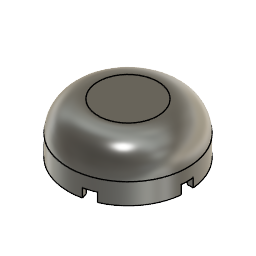
FlowerNubV0_v13 (Autodesk Fusion 360 design; units mm, degrees)
Autodesk Fusion 360 part; units mm, degrees
sketch "Sketch1" plane through (0, 0, 0) normal (0, 0, 1) x (1, 0, 0)
  circle A0 centre (0, 0) radius 3
  circle A1 centre (0, 0) radius 20
  dimension "d1" = 6
  dimension "d2" = 40
  constraint coincident A0.centre A1.centre
  constraint concentric A0 A1
  measures "d1" diameter of A0
  measures "d2" diameter of A1
extrude "Extrude1" add sketch "Sketch1" along normal blind 17 contours A0 | A1
fillet "Fillet1" radius 10 1 edges at (-18.6465, -7.2323, 17)
shell "Shell1" thickness 2 removed faces 1 at (4.7423, -7.1112, 0)
sketch "Sketch3" plane through (0, 0, 0) normal (0, 0, -1) x (1, 0, 0)
  circle A0 centre (0, 0) radius 18
  circle A1 centre (0, 0) radius 20
  line L0 (0, 0) -> (22, 0)
  line L1 (22, 0) -> (22, 2)
  line L2 (22, 0) -> (22, -2)
  line L3 (22, 2) -> (15, 2)
  line L4 (15, 2) -> (15, -2)
  line L5 (15, -2) -> (22, -2)
  line L6 (22, -2) -> (22, 2)
  line L7 (4.8963, 21.5413) -> (2.7331, 14.8839)
  line L8 (8.7005, 20.3052) -> (4.8963, 21.5413)
  line L9 (6.5374, 13.6478) -> (8.7005, 20.3052)
  line L10 (2.7331, 14.8839) -> (6.5374, 13.6478)
  line L11 (-18.9739, 11.3132) -> (-13.3108, 7.1987)
  line L12 (-16.6228, 14.5493) -> (-18.9739, 11.3132)
  line L13 (-10.9597, 10.4348) -> (-16.6228, 14.5493)
  line L14 (-13.3108, 7.1987) -> (-10.9597, 10.4348)
  line L15 (-16.6228, -14.5493) -> (-10.9597, -10.4348)
  line L16 (-18.9739, -11.3132) -> (-16.6228, -14.5493)
  line L17 (-13.3108, -7.1987) -> (-18.9739, -11.3132)
  line L18 (-10.9597, -10.4348) -> (-13.3108, -7.1987)
  line L19 (8.7005, -20.3052) -> (6.5374, -13.6478)
  line L20 (4.8963, -21.5413) -> (8.7005, -20.3052)
  line L21 (2.7331, -14.8839) -> (4.8963, -21.5413)
  line L22 (6.5374, -13.6478) -> (2.7331, -14.8839)
  dimension "d11" = 2
  dimension "d12" = 2
  dimension "d14" = 360
  constraint coincident A0.centre A1.centre
  constraint horizontal L0
  constraint perpendicular L0 L1
  constraint perpendicular L0 L2
  constraint horizontal L3
  constraint vertical L4
  constraint horizontal L5
  constraint vertical L6
  measures "d11" distance of L0.end L1.end
  measures "d12" distance of L0.end L2.end
extrude "Extrude3" cut sketch "Sketch3" against normal blind 3 contours A0 L0 L3 L4 | A0 A1 L0 L5 | A0 A1 L0 L3 | A0 L0 L4 L5 | A1 L0 L2 L5 L6 | A1 L0 L1 L3 L6 | A0 L7 L9 L10 | A0 A1 L7 L9 | A0 A1 L19 L21 | A0 L19 L21 L22 | A1 L7 L8 L9 | A1 L19 L20 L21 | A0 L11 L13 L14 | A0 A1 L11 L13 | A0 A1 L15 L17 | A0 L15 L17 L18 | A1 L11 L12 L13 | A1 L15 L16 L17
chamfer "Chamfer1" distance 2 angle 45 5 edges at (-14.5623, -10.5801, 3) (-14.5623, 10.5801, 3) (5.5623, 17.119, 3) (18, 0, 3) (5.5623, -17.119, 3) tangent chain off
sketch "Sketch2" plane through (0, 0, 15) normal (0, 0, -1) x (1, 0, 0)
  circle A0 centre (0, 0) radius 10
  circle A1 centre (0, 0) radius 3
  circle A2 centre (0, 0) radius 5
  line L0 (6.5, -1.25) -> (-6.5, -1.25)
  line L1 (-6.5, -1.25) -> (-6.5, 1.25)
  line L2 (-6.5, 1.25) -> (6.5, 1.25)
  line L3 (6.5, 1.25) -> (6.5, -1.25)
  line L4 (6.5, -1.25) -> (-6.5, 1.25) construction
  line L5 (-6.5, -1.25) -> (6.5, 1.25) construction
  dimension "d8" = 6
  dimension "d21" = 10
  dimension "d22" = 2.5
  constraint coincident A0.centre A1.centre
  constraint horizontal L0
  constraint perpendicular L0 L1
  constraint parallel L0 L2
  constraint parallel L1 L3
  constraint coincident L4 A0.centre
  constraint coincident L5 A0.centre
  measures "d8" diameter of A1
  measures "d21" diameter of A2
  measures "d22" distance of L0.end L1.end
extrude "Extrude5" add sketch "Sketch2" along normal blind 1 contours A1 L0 L2 | A1 A2 L0 L2 | A1 L2 | A1 L0 | A1 A2 L0 L2
extrude "Extrude6" cut sketch "Sketch2" against normal blind 1 contours A1 A2 L2 | A1 A2 L0
